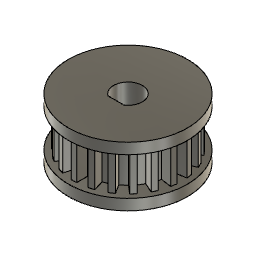
pulley2022 (Autodesk Fusion 360 design; units mm, degrees)
Autodesk Fusion 360 part; units mm, degrees
sketch "Sketch1" plane through (0, 0, 0) normal (0, 0, 1) x (1, 0, 0)
  line L0 (0, 0) -> (0, 10) construction
  line L1 (0.5, 8) -> (0.5, 10)
  line L2 (0.5, 10) -> (-0.5, 10)
  line L3 (-0.5, 10) -> (-0.5, 8)
  circle A0 centre (0, 0) radius 8.0156
  line L4 (-3.2971, 9.4541) -> (-2.7336, 7.5351)
  line L5 (-2.3376, 9.7358) -> (-3.2971, 9.4541)
  line L6 (-1.7741, 7.8168) -> (-2.3376, 9.7358)
  line L7 (-5.827, 8.1422) -> (-4.7458, 6.4597)
  line L8 (-4.9858, 8.6829) -> (-5.827, 8.1422)
  line L9 (-3.9045, 7.0003) -> (-4.9858, 8.6829)
  line L10 (-7.8849, 6.1707) -> (-6.3734, 4.861)
  line L11 (-7.2301, 6.9265) -> (-7.8849, 6.1707)
  line L12 (-5.7186, 5.6168) -> (-7.2301, 6.9265)
  line L13 (-9.304, 3.6993) -> (-7.4848, 2.8685)
  line L14 (-8.8886, 4.609) -> (-9.304, 3.6993)
  line L15 (-7.0693, 3.7781) -> (-8.8886, 4.609)
  line L16 (-9.9694, 0.9282) -> (-7.9897, 0.6436)
  line L17 (-9.8271, 1.9181) -> (-9.9694, 0.9282)
  line L18 (-7.8474, 1.6334) -> (-9.8271, 1.9181)
  line L19 (-9.8271, -1.9181) -> (-7.8474, -1.6334)
  line L20 (-9.9694, -0.9282) -> (-9.8271, -1.9181)
  line L21 (-7.9897, -0.6436) -> (-9.9694, -0.9282)
  line L22 (-8.8886, -4.609) -> (-7.0693, -3.7781)
  line L23 (-9.304, -3.6993) -> (-8.8886, -4.609)
  line L24 (-7.4848, -2.8685) -> (-9.304, -3.6993)
  line L25 (-7.2301, -6.9265) -> (-5.7186, -5.6168)
  line L26 (-7.8849, -6.1707) -> (-7.2301, -6.9265)
  line L27 (-6.3734, -4.861) -> (-7.8849, -6.1707)
  line L28 (-4.9858, -8.6829) -> (-3.9045, -7.0003)
  line L29 (-5.827, -8.1422) -> (-4.9858, -8.6829)
  line L30 (-4.7458, -6.4597) -> (-5.827, -8.1422)
  line L31 (-2.3376, -9.7358) -> (-1.7741, -7.8168)
  line L32 (-3.2971, -9.4541) -> (-2.3376, -9.7358)
  line L33 (-2.7336, -7.5351) -> (-3.2971, -9.4541)
  line L34 (0.5, -10) -> (0.5, -8)
  line L35 (-0.5, -10) -> (0.5, -10)
  line L36 (-0.5, -8) -> (-0.5, -10)
  line L37 (3.2971, -9.4541) -> (2.7336, -7.5351)
  line L38 (2.3376, -9.7358) -> (3.2971, -9.4541)
  line L39 (1.7741, -7.8168) -> (2.3376, -9.7358)
  line L40 (5.827, -8.1422) -> (4.7458, -6.4597)
  line L41 (4.9858, -8.6829) -> (5.827, -8.1422)
  line L42 (3.9045, -7.0003) -> (4.9858, -8.6829)
  line L43 (7.8849, -6.1707) -> (6.3734, -4.861)
  line L44 (7.2301, -6.9265) -> (7.8849, -6.1707)
  line L45 (5.7186, -5.6168) -> (7.2301, -6.9265)
  line L46 (9.304, -3.6993) -> (7.4848, -2.8685)
  line L47 (8.8886, -4.609) -> (9.304, -3.6993)
  line L48 (7.0693, -3.7781) -> (8.8886, -4.609)
  line L49 (9.9694, -0.9282) -> (7.9897, -0.6436)
  line L50 (9.8271, -1.9181) -> (9.9694, -0.9282)
  line L51 (7.8474, -1.6334) -> (9.8271, -1.9181)
  line L52 (9.8271, 1.9181) -> (7.8474, 1.6334)
  line L53 (9.9694, 0.9282) -> (9.8271, 1.9181)
  line L54 (7.9897, 0.6436) -> (9.9694, 0.9282)
  line L55 (8.8886, 4.609) -> (7.0693, 3.7781)
  line L56 (9.304, 3.6993) -> (8.8886, 4.609)
  line L57 (7.4848, 2.8685) -> (9.304, 3.6993)
  line L58 (7.2301, 6.9265) -> (5.7186, 5.6168)
  line L59 (7.8849, 6.1707) -> (7.2301, 6.9265)
  line L60 (6.3734, 4.861) -> (7.8849, 6.1707)
  line L61 (-1.4773, -2.2) -> (1.4773, -2.2)
  arc A1 (1.4773, -2.2) -> (-1.4773, -2.2) centre (0, 0) ccw
  circle A2 centre (0, 0) radius 11
  line L62 (4.9858, 8.6829) -> (3.9045, 7.0003)
  line L63 (5.827, 8.1422) -> (4.9858, 8.6829)
  line L64 (4.7458, 6.4597) -> (5.827, 8.1422)
  line L65 (2.3376, 9.7358) -> (1.7741, 7.8168)
  line L66 (3.2971, 9.4541) -> (2.3376, 9.7358)
  line L67 (2.7336, 7.5351) -> (3.2971, 9.4541)
  dimension "d1" = 10
  dimension "d2" = 1
  dimension "d4" = 2
  dimension "d6" = 360
  dimension "d9" = 5.3
  dimension "d10" = 2.2
  dimension "d11" = 22
  constraint coincident L0.start A0.centre
  constraint vertical L0
  constraint vertical L1
  constraint horizontal L2
  constraint vertical L3
  constraint coincident L0.end L2
  constraint symmetric L0 L1 L3
  constraint coincident L1.start A0
  constraint coincident L3.end A0
  constraint horizontal L61
  measures "d1" distance of L0.start L2
  measures "d2" distance of L1 L3
  measures "d4" distance of L3.end L2.end
  measures "d9" diameter of A1
  measures "d10" distance of L0.start L61
  measures "d11" diameter of A2
extrude "Extrude1" add sketch "Sketch1" along normal blind 11 contours L1 L2 L3 A0 | A0 | A0 L65 L66 L67 | A0 L4 L5 L6 | A0 L62 L63 L64 | A0 L7 L8 L9 | A0 L58 L59 L60 | A0 L10 L11 L12 | A0 L55 L56 L57 | A0 L13 L14 L15 | A0 L52 L53 L54 | A0 L16 L17 L18 | A0 L49 L50 L51 | A0 L19 L20 L21 | A0 L46 L47 L48 | A0 L22 L23 L24 | A0 L43 L44 L45 | A0 L25 L26 L27 | A0 L40 L41 L42 | A0 L28 L29 L30 | A0 L37 L38 L39 | A0 L31 L32 L33 | A0 L34 L35 L36
extrude "Extrude2" add sketch "Sketch1" along normal blind 2 contours A0 | A2
extrude "Extrude3" add sketch "Sketch1" against normal blind 2 from surface at 11 contours A0 | A2
